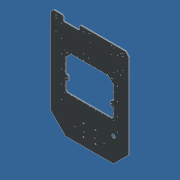
# Autodesk Inventor part: Husky_top_plate
Saved by Autodesk Inventor 2016 (Build 200138000, 138)
## iProperties
Created: 2021-06-09
Part Number: Husky_top_plate
Material: Generico
Document SubType Name: Modeling
Designer: Galli Davide
Density: 1 g/cm^3
Appearance: Grigio ferro
Author: Galli Davide
Autodesk Inventor part; units mm, degrees
ref_plane "YZ Plane" through (0, 0, 0) normal (1, 0, 0) x (0, 1, 0)
ref_plane "XZ Plane" through (0, 0, 0) normal (0, 1, 0) x (-1, 0, 0)
ref_plane "XY Plane" through (0, 0, 0) normal (0, 0, 1) x (1, 0, 0)
sketch "Schizzo1" plane through (0, 0, 0) normal (0, 1, 0) x (-1, 0, 0)
  line L0 (0, 0) -> (620, 0)
  line L1 (620, 0) -> (620, -820)
  line L2 (620, -820) -> (0, -820)
  line L3 (0, -820) -> (0, 0)
  dimension "d0" = 620
  dimension "d1" = 820
  constraints: 8 end point, 2 parallel, 1 horizontal, 1 perpendicular
  measures "d0" distance of L1.end L2.end
  measures "d1" distance of L0.end L1.end
extrude "Estrusione1" add sketch "Schizzo1" along normal blind 8
chamfer "Smusso1" distance 120 angle 45 2 edges at (0, 4, -820) (-620, 4, -820)
chamfer "Smusso2" distance 25 angle 45 2 edges at (-620, 4, 0) (0, 4, 0)
sketch "Schizzo2" plane through (0, 8, 0) normal (0, 1, 0) x (1, 0, 0)
  line L0 (-520, 0) -> (-390, 0)
  line L1 (-390, 0) -> (-390, 40)
  line L2 (-390, 40) -> (-520, 40)
  line L3 (-520, 40) -> (-520, 0)
  line L4 (-620, 700) -> (-620, 25) projected
  point P0 (0, 0)
  dimension "d10" = 130
  dimension "d11" = 40
  dimension "d12" = 100
  constraints: 8 end point, 2 parallel, 1 horizontal, 1 perpendicular
  measures "d10" distance of L2.end L1.end
  measures "d11" distance of L1.end L0.end
  measures "d12" distance between parallel lines of L4 L3
extrude "Estrusione2" cut sketch "Schizzo2" against normal blind 8
fillet "Raccordo1" radius 10 4 edges at (-390, 4, 0) (-390, 4, -40) (-520, 4, 0) (-520, 4, -40)
sketch "Schizzo3" plane through (0, 8, 0) normal (0, 1, 0) x (1, 0, 0)
  line L0 (-120, 820) -> (-500, 820) projected
  line L1 (0, 25) -> (0, 700) projected
  line L2 (-380, 0) -> (-25, 0) projected
  line L3 (-310, 820) -> (-310, 0) construction
  circle A0 centre (-120, 630) radius 15
  point P0 (0, 0)
  point P1 (-86.5, 60)
  point P2 (-86.5, 165)
  point P3 (-86.5, 270)
  point P4 (-86.5, 375)
  point P5 (-86.5, 480)
  point P6 (-86.5, 585)
  point P7 (-533.5, 60)
  point P8 (-533.5, 165)
  point P9 (-533.5, 270)
  point P10 (-533.5, 375)
  point P11 (-533.5, 480)
  point P12 (-533.5, 585)
  dimension "d16" = 190
  dimension "d17" = 120
  dimension "d18" = 86.5
  dimension "d21" = 105
  dimension "d26" = 60
  dimension "d27" = 30
  constraints: 6 symmetric about line, 2 end point, 1 centre point, 1 coincident, 1 midpoint, 1 perpendicular, 1 point on line, 1 vertical, 5 other
  measures "d16" distance from line of L0 point (-120, 630)
  measures "d17" distance from line of L1 point (-120, 630)
  measures "d18" distance from line of L1 point (-86.5, 60)
  measures "d21" distance of point (-86.5, 60) point (-86.5, 165)
  measures "d26" distance from line of L2 point (-86.5, 60)
  measures "d27" diameter of A0
extrude "Estrusione3" cut sketch "Schizzo3" against normal blind 8
hole "Foro1" at (-120, 8, -630) at (-86.5, 8, -60) at (-86.5, 8, -165) at (-86.5, 8, -270) at (-86.5, 8, -375) at (-86.5, 8, -480) at (-86.5, 8, -585) at (-533.5, 8, -585) at (-533.5, 8, -480) at (-533.5, 8, -375) at (-533.5, 8, -270) at (-533.5, 8, -165) at (-533.5, 8, -60) direction (0, -1, 0) diameter 5 end through all
sketch "Schizzo4" plane through (0, 8, 0) normal (0, 1, 0) x (1, 0, 0)
  line L0 (-120, 820) -> (-500, 820) projected
  line L1 (0, 25) -> (0, 700) projected
  line L2 (-500, 820) -> (-120, 820) projected
  line L3 (-310, 820) -> (-310, 0) construction
  line L4 (-25, 0) -> (-380, 0) projected
  point P0 (0, 0)
  point P1 (-195, 717.5)
  point P2 (-267, 717.5)
  point P3 (-425, 717.5)
  point P4 (-353, 717.5)
  dimension "d37" = 72
  dimension "d38" = 102.5
  dimension "d39" = 195
  constraints: 2 end point, 2 symmetric about line, 1 horizontal alignment, 1 midpoint, 1 point on line, 1 vertical
  measures "d37" distance of point (-195, 717.5) point (-267, 717.5)
  measures "d38" distance from line of L0 point (-195, 717.5)
  measures "d39" distance from line of L1 point (-195, 717.5)
hole "Foro2" at (-195, 8, -717.5) at (-267, 8, -717.5) at (-425, 8, -717.5) at (-353, 8, -717.5) direction (0, -1, 0) diameter 5 end through all countersink diameter 10 countersink angle 45
sketch "Schizzo5" plane through (0, 8, 0) normal (0, 1, 0) x (1, 0, 0)
  line L0 (-120, 820) -> (-500, 820) projected
  line L1 (0, 25) -> (0, 700) projected
  line L2 (-500, 820) -> (-120, 820) projected
  line L3 (-310, 820) -> (-310, 545.1778) construction
  point P0 (0, 0)
  point P1 (-262.5, 755)
  point P2 (-357.5, 755)
  point P3 (-262.5, 660)
  point P4 (-357.5, 660)
  dimension "d47" = 65
  dimension "d50" = 95
  dimension "d53" = 95
  dimension "d56" = 47.5
  constraints: 2 end point, 2 vertical, 1 horizontal, 1 midpoint, 3 other
  measures "d47" distance from line of L0 point (-262.5, 755)
  measures "d50" distance of point (-262.5, 755) point (-357.5, 755)
  measures "d53" distance of point (-262.5, 755) point (-262.5, 660)
  measures "d56" distance from line of L3 point (-262.5, 755)
hole "Foro3" at (-262.5, 8, -755) at (-357.5, 8, -755) at (-262.5, 8, -660) at (-357.5, 8, -660) direction (0, -1, 0) diameter 10 end through all
sketch "Schizzo6" plane through (0, 8, 0) normal (0, 1, 0) x (1, 0, 0)
  line L0 (-122.5, 515) -> (-497.5, 515)
  line L1 (-497.5, 235) -> (-122.5, 235)
  line L2 (-120, 820) -> (-500, 820) projected
  line L3 (-497.5, 433) -> (-477.5, 433)
  line L4 (-477.5, 433) -> (-477.5, 393)
  line L5 (-477.5, 393) -> (-497.5, 393)
  line L6 (-310, 515) -> (-310, 447.5629) construction
  line L7 (-122.5, 433) -> (-142.5, 433)
  line L8 (-142.5, 433) -> (-142.5, 393)
  line L9 (-142.5, 393) -> (-122.5, 393)
  line L10 (-497.5, 515) -> (-497.5, 433)
  line L11 (-497.5, 393) -> (-497.5, 235)
  line L12 (-122.5, 235) -> (-122.5, 393)
  line L13 (-122.5, 433) -> (-122.5, 515)
  point P0 (0, 0)
  point P1 (-310, 820)
  dimension "d64" = 375
  dimension "d65" = 280
  dimension "d66" = 305
  dimension "d69" = 82
  dimension "d71" = 40
  dimension "d72" = 20
  constraints: 26 end point, 6 parallel, 4 symmetric about line, 3 perpendicular, 2 horizontal, 2 midpoint, 1 vertical, 1 vertical alignment
  measures "d64" distance of L0.start L0.end
  measures "d65" distance of L1.end L0.start
  measures "d66" distance between parallel lines of L2 L0
  measures "d69" distance between parallel lines of L0 L3
  measures "d71" distance of L3.end L4.end
  measures "d72" distance of L4.end L5.end
extrude "Estrusione4" cut sketch "Schizzo6" against normal blind 8
chamfer "Smusso3" distance 10 angle 45 2 edges at (-497.5, 4, -515) (-122.5, 4, -515)
chamfer "Smusso4" distance 40 angle 45 2 edges at (-497.5, 4, -235) (-122.5, 4, -235)
chamfer "Smusso5" distance 5 angle 45 8 edges at (-122.5, 4, -433) (-142.5, 4, -433) (-142.5, 4, -393) (-122.5, 4, -393) (-497.5, 4, -433) (-477.5, 4, -433) (-477.5, 4, -393) (-497.5, 4, -393)
sketch "Schizzo7" plane through (0, 8, 0) normal (0, 1, 0) x (1, 0, 0)
  line L0 (-477.5, 398) -> (-477.5, 428) projected
  line L1 (-482.5, 433) -> (-492.5, 433) projected
  line L2 (-127.5, 433) -> (-137.5, 433) projected
  line L3 (-142.5, 428) -> (-142.5, 398) projected
  point P0 (0, 0)
  point P1 (-487.5, 413)
  point P2 (-132.5, 413)
  point P3 (-132.5, 240)
  point P4 (-487.5, 240)
  dimension "d84" = 173
  dimension "d85" = 10
  dimension "d86" = 20
  dimension "d87" = 20
  dimension "d88" = 10
  constraints: 2 horizontal alignment, 2 vertical alignment
  measures "d84" distance of point (-487.5, 240) point (-487.5, 413)
  measures "d85" distance from line of L0 point (-487.5, 413)
  measures "d86" distance from line of L1 point (-487.5, 413)
  measures "d87" distance from line of L2 point (-132.5, 413)
  measures "d88" distance from line of L3 point (-132.5, 413)
hole "Foro4" at (-487.5, 8, -413) at (-132.5, 8, -413) at (-132.5, 8, -240) at (-487.5, 8, -240) direction (0, -1, 0) diameter 7 end through all countersink diameter 14 countersink angle 45
sketch "Schizzo8" plane through (0, 8, 0) normal (0, 1, 0) x (1, 0, 0)
  line L0 (-122.5, 515) -> (-497.5, 515) construction
  line L1 (-497.5, 515) -> (-497.5, 235) construction
  line L2 (-497.5, 235) -> (-122.5, 235) construction
  line L3 (-122.5, 235) -> (-122.5, 515) construction
  line L4 (-503.5, 521) -> (-116.5, 521) construction
  line L5 (-116.5, 521) -> (-116.5, 229) construction
  line L6 (-116.5, 229) -> (-503.5, 229) construction
  line L7 (-503.5, 229) -> (-503.5, 521) construction
  point P0 (0, 0)
  point P1 (-164.875, 521)
  point P2 (-213.25, 521)
  point P3 (-261.625, 521)
  point P4 (-310, 521)
  point P5 (-358.375, 521)
  point P6 (-406.75, 521)
  point P7 (-455.125, 521)
  point P8 (-503.5, 521)
  point P9 (-116.5, 229)
  point P10 (-164.875, 229)
  point P11 (-213.25, 229)
  point P12 (-261.625, 229)
  point P13 (-310, 229)
  point P14 (-358.375, 229)
  point P15 (-406.75, 229)
  point P16 (-455.125, 229)
  point P17 (-503.5, 229)
  point P18 (-116.5, 277.6667)
  point P19 (-116.5, 326.3333)
  point P20 (-116.5, 375)
  point P21 (-116.5, 423.6667)
  point P22 (-116.5, 472.3333)
  point P23 (-503.5, 277.6667)
  point P24 (-503.5, 326.3333)
  point P25 (-503.5, 375)
  point P26 (-503.5, 423.6667)
  point P27 (-503.5, 472.3333)
  dimension "d96" = 375
  dimension "d97" = 280
  dimension "d98" = 6
  dimension "d99" = 387
  dimension "d100" = 292
  dimension "d103" = 48.375
  dimension "d106" = 292
  dimension "d114" = 48.6667
  dimension "d118" = 48.6667
  constraints: 16 end point, 4 parallel, 3 vertical, 2 horizontal, 2 perpendicular, 1 coincident, 30 other
  measures "d96" distance of L2.end L1.end
  measures "d97" distance of L1.end L0.end
  measures "d98" distance between parallel lines of L0 L4
  measures "d99" distance of L4.start L4.end
  measures "d100" distance of L4.end L5.end
  measures "d103" distance of point (-116.5, 521) point (-164.875, 521)
  measures "d106" distance of point (-116.5, 521) point (-116.5, 229)
  measures "d114" distance of point (-116.5, 229) point (-116.5, 277.667)
  measures "d118" distance of point (-503.5, 229) point (-503.5, 277.667)
hole "Foro5" at (-116.5, 8, -521) at (-164.875, 8, -521) at (-213.25, 8, -521) at (-261.625, 8, -521) at (-310, 8, -521) at (-358.375, 8, -521) at (-406.75, 8, -521) at (-455.125, 8, -521) at (-503.5, 8, -521) at (-116.5, 8, -229) at (-164.875, 8, -229) at (-213.25, 8, -229) at (-261.625, 8, -229) at (-310, 8, -229) at (-358.375, 8, -229) at (-406.75, 8, -229) at (-455.125, 8, -229) at (-503.5, 8, -229) at (-116.5, 8, -277.6667) at (-116.5, 8, -326.3333) at (-116.5, 8, -375) at (-116.5, 8, -423.6667) at (-116.5, 8, -472.3333) at (-503.5, 8, -277.6667) at (-503.5, 8, -326.3333) at (-503.5, 8, -375) at (-503.5, 8, -423.6667) at (-503.5, 8, -472.3333) direction (0, -1, 0) diameter 3.459 end through all thread size "M4x0.5" class "6H" standard "ISO Metric profile"
sketch "Schizzo9" plane through (0, 8, 0) normal (0, 1, 0) x (1, 0, 0)
  line L0 (-380, 0) -> (-25, 0) projected
  line L1 (0, 25) -> (0, 700) projected
  line L2 (-500, 820) -> (-120, 820) projected
  line L3 (-310, 820) -> (-310, 614.2026) construction
  point P0 (0, 0)
  point P1 (-45, 45)
  point P2 (-45, 25)
  point P3 (-575, 45)
  point P4 (-575, 25)
  dimension "d130" = 20
  dimension "d131" = 25
  dimension "d132" = 45
  constraints: 2 end point, 2 symmetric about line, 1 midpoint, 1 vertical, 1 vertical alignment
  measures "d130" distance of point (-45, 25) point (-45, 45)
  measures "d131" distance from line of L0 point (-45, 25)
  measures "d132" distance from line of L1 point (-45, 45)
hole "Foro6" at (-45, 8, -45) at (-45, 8, -25) at (-575, 8, -45) at (-575, 8, -25) direction (0, -1, 0) diameter 5 end through all
sketch "Schizzo10" plane through (0, 8, 0) normal (0, 1, 0) x (1, 0, 0)
  line L0 (-620, 700) -> (-620, 25) projected
  line L1 (-595, 0) -> (-530, 0) projected
  line L2 (-310, 820) -> (-310, 614.2026) construction
  point P0 (0, 0)
  point P1 (-575, 140)
  point P2 (-45, 140)
  dimension "d140" = 45
  dimension "d141" = 140
  constraints: 1 symmetric about line
  measures "d140" distance from line of L0 point (-575, 140)
  measures "d141" distance from line of L1 point (-575, 140)
hole "Foro7" at (-575, 8, -140) at (-45, 8, -140) direction (0, -1, 0) diameter 3.459 end through all thread size "M4x0.5" class "6H" standard "ISO Metric profile"
sketch "Schizzo11" plane through (0, 8, 0) normal (0, 1, 0) x (1, 0, 0)
  line L0 (-380, 0) -> (-25, 0) projected
  line L1 (0, 25) -> (0, 700) projected
  point P0 (0, 0)
  point P1 (-300, 75)
  point P2 (-300, 15)
  point P3 (-135, 15)
  point P4 (-135, 75)
  dimension "d149" = 15
  dimension "d150" = 75
  dimension "d151" = 165
  dimension "d152" = 135
  constraints: 2 horizontal alignment, 2 vertical alignment
  measures "d149" distance from line of L0 point (-135, 15)
  measures "d150" distance from line of L0 point (-135, 75)
  measures "d151" distance of point (-135, 75) point (-300, 75)
  measures "d152" distance from line of L1 point (-135, 75)
hole "Foro8" at (-135, 8, -15) at (-135, 8, -75) at (-300, 8, -75) at (-300, 8, -15) direction (0, -1, 0) diameter 3.459 end through all thread size "M4x0.5" class "6H" standard "ISO Metric profile"
sketch "Schizzo12" plane through (0, 8, 0) normal (0, 1, 0) x (1, 0, 0)
  line L0 (-380, 0) -> (-25, 0) projected
  line L1 (0, 25) -> (0, 700) projected
  point P0 (0, 0)
  point P1 (-316, 22)
  point P2 (-316, 192)
  point P3 (-116, 192)
  point P4 (-116, 22)
  dimension "d161" = 22
  dimension "d162" = 116
  dimension "d163" = 200
  dimension "d164" = 170
  constraints: 2 horizontal alignment, 2 vertical alignment
  measures "d161" distance from line of point (-116, 22) L0
  measures "d162" distance from line of L1 point (-116, 192)
  measures "d163" distance of point (-316, 192) point (-116, 192)
  measures "d164" distance of point (-116, 22) point (-116, 192)
hole "Foro9" at (-316, 8, -192) at (-116, 8, -192) at (-116, 8, -22) at (-316, 8, -22) direction (0, -1, 0) diameter 3.459 end through all thread size "M4x0.5" class "6H" standard "ISO Metric profile"
sketch "Schizzo13" plane through (0, 8, 0) normal (0, 1, 0) x (1, 0, 0)
  line L0 (0, 25) -> (0, 700) projected
  line L1 (-380, 0) -> (-25, 0) projected
  point P0 (0, 0)
  point P1 (-359, 183)
  point P2 (-359, 33)
  point P3 (-64, 33)
  point P4 (-64, 183)
  dimension "d172" = 295
  dimension "d173" = 150
  dimension "d174" = 64
  dimension "d175" = 183
  constraints: 2 horizontal alignment, 2 vertical alignment
  measures "d172" distance of point (-64, 183) point (-359, 183)
  measures "d173" distance of point (-64, 33) point (-64, 183)
  measures "d174" distance from line of L0 point (-64, 183)
  measures "d175" distance from line of point (-64, 183) L1
hole "Foro10" at (-359, 8, -183) at (-359, 8, -33) at (-64, 8, -183) at (-64, 8, -33) direction (0, -1, 0) diameter 4.459 end through all thread size "M5x0.5" class "6H" standard "ISO Metric profile"
equation "\"d56\" = 0.5 * d50"
equation "\"d103\" = 0.125 * d99"
equation "\"d106\" = d100"
equation "\"d114\" = 0.166667 * d100"
equation "\"d118\" = 0.166667 * d100"
